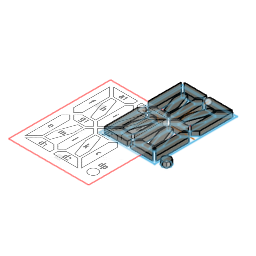
16 Seg Digit v1 (Autodesk Fusion 360 design; units mm, degrees)
Autodesk Fusion 360 part; units mm, degrees
sketch "Sketch1" plane through (0, 0, 0) normal (0, 0, 1) x (1, 0, 0)
  line L0 (0.7992, 17.6925) -> (5.7249, 17.6925)
  line L1 (5.7249, 17.6925) -> (5.7249, 16.8295)
  line L2 (5.7249, 16.8295) -> (4.8548, 15.8682)
  line L3 (4.8548, 15.8682) -> (2.6095, 15.8682)
  line L4 (2.6095, 15.8682) -> (0.7992, 17.6925)
  line L5 (6.0446, 16.5847) -> (6.0446, 17.6925) construction
  line L6 (5.5548, 9.0271) -> (6.5259, 9.0271) construction
  line L7 (6.5259, 9.0271) -> (6.7604, 9.0271) construction
  line L8 (6.7604, 9.0271) -> (11.6566, 9.0271) construction
  line L9 (6.0446, 16.5847) -> (6.0446, 17.6925) construction
  line L10 (11.29, 17.6925) -> (6.3643, 17.6925)
  line L11 (9.4797, 15.8682) -> (11.29, 17.6925)
  line L12 (6.3643, 17.6925) -> (6.3643, 16.8295)
  line L13 (6.3643, 16.8295) -> (7.2344, 15.8682)
  line L14 (7.2344, 15.8682) -> (9.4797, 15.8682)
  line L15 (2.5728, 15.6182) -> (3.6447, 15.6182)
  line L16 (3.6447, 15.6182) -> (4.8536, 12.233)
  line L17 (4.8536, 12.233) -> (4.8536, 10.2469)
  line L18 (4.8536, 10.2469) -> (3.8002, 10.2469)
  line L19 (3.8002, 10.2469) -> (2.5519, 13.5834)
  line L20 (2.5519, 13.5834) -> (2.5728, 15.6182)
  line L21 (0.463, 17.3791) -> (2.2782, 15.6012)
  line L22 (2.2782, 15.6012) -> (2.2782, 10.188)
  line L23 (2.2782, 10.188) -> (1.3706, 9.2613)
  line L24 (1.3706, 9.2613) -> (0.4244, 10.188)
  line L25 (0.4244, 10.188) -> (0.4244, 17.4168)
  line L26 (0.4244, 17.4168) -> (0.463, 17.3791)
  line L27 (5.1451, 10.2118) -> (5.1451, 15.6233)
  line L28 (6.9441, 15.6233) -> (6.9441, 10.2118)
  line L29 (6.9441, 10.2118) -> (5.1451, 15.6233) construction
  line L30 (5.1451, 10.2118) -> (6.9441, 15.6233) construction
  line L31 (5.1451, 10.2118) -> (6.0446, 9.3447)
  line L32 (6.0446, 9.3447) -> (6.9441, 10.2118)
  line L33 (5.1451, 15.6233) -> (6.0446, 16.4904)
  line L34 (6.9441, 15.6233) -> (6.0446, 16.4904)
  line L35 (4.8772, 9.943) -> (2.581, 9.943)
  line L36 (2.581, 8.1112) -> (4.8772, 8.1112)
  line L37 (4.8772, 9.943) -> (2.581, 8.1112) construction
  line L38 (2.581, 9.943) -> (4.8772, 8.1112) construction
  line L39 (2.581, 9.943) -> (1.7172, 9.0271)
  line L40 (2.581, 8.1112) -> (1.7172, 9.0271)
  line L41 (4.8772, 8.1112) -> (5.741, 9.0271)
  line L42 (4.8772, 9.943) -> (5.741, 9.0271)
  line L43 (11.6566, 9.0271) -> (5.741, 9.0271) construction
  line L44 (1.7172, 9.0271) -> (0.325, 9.0271) construction
  line L45 (7.2369, 8.1112) -> (6.3731, 9.0271)
  line L46 (7.2369, 8.1112) -> (9.5331, 8.1112)
  line L47 (9.5331, 8.1112) -> (10.3968, 9.0271)
  line L48 (9.5331, 9.943) -> (10.3968, 9.0271)
  line L49 (9.5331, 9.943) -> (7.2369, 9.943)
  line L50 (7.2369, 9.943) -> (6.3731, 9.0271)
  line L51 (6.9441, 7.8337) -> (6.9441, 2.4221)
  line L52 (6.9441, 7.8337) -> (6.0446, 8.7008)
  line L53 (5.1451, 7.8337) -> (6.0446, 8.7008)
  line L54 (5.1451, 2.4221) -> (5.1451, 7.8337)
  line L55 (5.1451, 2.4221) -> (6.0446, 1.555)
  line L56 (6.0446, 1.555) -> (6.9441, 2.4221)
  line L57 (4.8536, 7.8074) -> (3.8002, 7.8074)
  line L58 (3.8002, 7.8074) -> (2.5519, 4.4709)
  line L59 (2.5519, 4.4709) -> (2.5728, 2.436)
  line L60 (2.5728, 2.436) -> (3.6447, 2.436)
  line L61 (3.6447, 2.436) -> (4.8536, 5.8212)
  line L62 (4.8536, 5.8212) -> (4.8536, 7.8074)
  line L63 (8.289, 10.2469) -> (9.5373, 13.5834)
  line L64 (9.5373, 13.5834) -> (9.5164, 15.6182)
  line L65 (9.5164, 15.6182) -> (8.4444, 15.6182)
  line L66 (8.4444, 15.6182) -> (7.2356, 12.233)
  line L67 (7.2356, 12.233) -> (7.2356, 10.2469)
  line L68 (7.2356, 10.2469) -> (8.289, 10.2469)
  line L69 (8.289, 7.8074) -> (9.5373, 4.4709)
  line L70 (9.5373, 4.4709) -> (9.5164, 2.436)
  line L71 (9.5164, 2.436) -> (8.4444, 2.436)
  line L72 (8.4444, 2.436) -> (7.2356, 5.8212)
  line L73 (7.2356, 7.8074) -> (8.289, 7.8074)
  line L74 (7.2356, 5.8212) -> (7.2356, 7.8074)
  line L75 (6.3643, 0.3617) -> (6.3643, 1.2248)
  line L76 (6.3643, 1.2248) -> (7.2344, 2.186)
  line L77 (7.2344, 2.186) -> (9.4797, 2.186)
  line L78 (11.29, 0.3617) -> (6.3643, 0.3617)
  line L79 (9.4797, 2.186) -> (11.29, 0.3617)
  line L80 (2.6095, 2.186) -> (0.7992, 0.3617)
  line L81 (0.7992, 0.3617) -> (5.7249, 0.3617)
  line L82 (5.7249, 0.3617) -> (5.7249, 1.2248)
  line L83 (4.8548, 2.186) -> (2.6095, 2.186)
  line L84 (5.7249, 1.2248) -> (4.8548, 2.186)
  line L85 (1.3706, 8.7929) -> (0.4244, 7.8662)
  line L86 (0.4244, 7.8662) -> (0.4244, 0.6374)
  line L87 (0.463, 0.6751) -> (2.2782, 2.4531)
  line L88 (2.2782, 7.8662) -> (1.3706, 8.7929)
  line L89 (2.2782, 2.4531) -> (2.2782, 7.8662)
  line L90 (0.4244, 0.6374) -> (0.463, 0.6751)
  line L91 (10.7186, 9.2613) -> (11.6647, 10.188)
  line L92 (11.6647, 10.188) -> (11.6647, 17.4168)
  line L93 (11.6647, 17.4168) -> (11.6262, 17.3791)
  line L94 (11.6262, 17.3791) -> (9.8109, 15.6012)
  line L95 (9.8109, 10.188) -> (10.7186, 9.2613)
  line L96 (9.8109, 15.6012) -> (9.8109, 10.188)
  line L97 (11.6647, 7.8662) -> (11.6647, 0.6374)
  line L98 (11.6647, 0.6374) -> (11.6262, 0.6751)
  line L99 (11.6262, 0.6751) -> (9.8109, 2.4531)
  line L100 (9.8109, 2.4531) -> (9.8109, 7.8662)
  line L101 (10.7186, 8.7929) -> (11.6647, 7.8662)
  line L102 (9.8109, 7.8662) -> (10.7186, 8.7929)
  line L103 (14.263, 1.2968) -> (13.9901, 1.9557)
  line L104 (13.9901, 1.9557) -> (13.3313, 2.2286)
  line L105 (13.3313, 2.2286) -> (12.6724, 1.9557)
  line L106 (12.6724, 1.9557) -> (12.3995, 1.2968)
  line L107 (12.3995, 1.2968) -> (12.6724, 0.638)
  line L108 (12.6724, 0.638) -> (13.3313, 0.3651)
  line L109 (13.3313, 0.3651) -> (13.9901, 0.638)
  line L110 (13.9901, 0.638) -> (14.263, 1.2968)
  point P0 (13.3313, 1.2968)
  constraint horizontal L0
  constraint perpendicular L0 L1
  constraint perpendicular L1 L3
  constraint perpendicular L0 L5
  constraint horizontal L15
  constraint perpendicular L15 L17
  constraint perpendicular L17 L18
  constraint vertical L22
  constraint perpendicular L21 L23
  constraint perpendicular L23 L24
  constraint parallel L22 L25
  constraint parallel L21 L26
  constraint parallel L27 L28
  constraint coincident L39.end L43
  constraint coincident L6 L41.end
  constraint horizontal L35
  constraint parallel L35 L36
  constraint horizontal L49
  constraint parallel L46 L49
  constraint parallel L51 L54
  constraint parallel L87 L90
extrude "Extrude1" add sketch "Sketch1" along normal blind 1 contours L103 L104 L105 L106 L107 L108 L109 L110 makes body 1
extrude "Extrude2" add sketch "Sketch1" along normal blind 1 separate body contours L0 L1 L2 L3 L4 | L10 L11 L12 L13 L14 | L15 L16 L17 L18 L19 L20 | L21 L22 L23 L24 L25 L26 | L27 L28 L31 L32 L33 L34 | L35 L36 L39 L40 L41 L42 | L45 L46 L47 L48 L49 L50 | L51 L52 L53 L54 L55 L56 | L57 L58 L59 L60 L61 L62 | L63 L64 L65 L66 L67 L68 | L69 L70 L71 L72 L73 L74 | L75 L76 L77 L78 L79 | L80 L81 L82 L83 L84 | L85 L86 L87 L88 L89 L90 | L91 L92 L93 L94 L95 L96 | L97 L98 L99 L100 L101 L102 makes body 2 at (1.0424, 3.6522, 0) makes body 3 at (8.4058, 4.2427, 0) makes body 4 at (3.0445, 17.0844, 0) makes body 5 at (11.0468, 14.402, 0) makes body 6 at (9.0447, 17.0844, 0) makes body 7 at (3.6834, 13.8115, 0) makes body 8 at (5.7448, 4.226, 0) makes body 9 at (3.0445, 0.9698, 0) makes body 10 at (3.6834, 4.2427, 0) makes body 11 at (8.7677, 9.3324, 0) makes body 12 at (5.7448, 13.8195, 0) makes body 13 at (11.0468, 3.6522, 1) makes body 14 at (8.4058, 13.8115, 0) makes body 15 at (1.0424, 14.402, 0) makes body 16 at (3.3464, 9.3324, 0) makes body 17 at (9.0447, 0.9698, 0)
sketch "Sketch2" plane through (0, 0, 0) normal (0, 0, 1) x (1, 0, 0)
  line L0 (0.0095, 0.0195) -> (12.0095, 0.0195)
  line L1 (12.0095, 0.0195) -> (12.0095, 18.0195)
  line L2 (12.0095, 18.0195) -> (0.0095, 18.0195)
  line L3 (0.0095, 18.0195) -> (0.0095, 0.0195)
  dimension "d5" = 12
  dimension "d6" = 18
  constraint horizontal L0
  constraint vertical L1
  constraint horizontal L2
  constraint vertical L3
  measures "d5" distance of L0.start L0.end
  measures "d6" distance of L0.start L2.end
named bodies: "Point", "LeftDown", "Diagonal DR", "TopLeft", "RightTop", "TopRight", "Diagonal TL", "Down", "DownLeft", "Diagonal DL", "Right", "Top", "RightDown", "Diagonal TR", "LeftTop", "Left", "DownRight"
